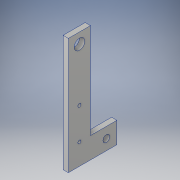
# Autodesk Inventor part: PaddleCollection2.1AxleSupport
Saved by Autodesk Inventor 2019 (Build 230136000, 136)
## iProperties
Created: 2018-10-20
Part Number: PaddleCollection2.1AxleSupport
Material: Aluminum 6061
Document SubType Name: Modeling
Designer: User
Density: 2.7 g/cm^3
Appearance: Aluminum - Flat
Author: User
Autodesk Inventor part; units mm, degrees
ref_plane "YZ Plane" through (0, 0, 0) normal (1, 0, 0) x (0, 1, 0)
ref_plane "XZ Plane" through (0, 0, 0) normal (0, 1, 0) x (-1, 0, 0)
ref_plane "XY Plane" through (0, 0, 0) normal (0, 0, 1) x (1, 0, 0)
sketch "Sketch1" plane through (0, 0, 0) normal (1, 0, 0) x (0, 1, 0)
  line L0 (0, 0) -> (139.7, 0)
  line L1 (139.7, 0) -> (139.7, -58.2676)
  line L2 (139.7, -58.2676) -> (0, -58.2676)
  line L3 (0, -58.2676) -> (0, 0)
  circle A0 centre (127, -13.2588) radius 6.35
  circle A1 centre (12.7, -45.5676) radius 4.064
  line L4 (139.7, -58.2676) -> (25.4, -58.2676)
  line L5 (25.4, -58.2676) -> (25.4, -26.5176)
  line L6 (25.4, -26.5176) -> (139.7, -26.5176)
  line L7 (139.7, -26.5176) -> (139.7, -58.2676)
  dimension "d0" = 139.7
  dimension "d2" = 12.7
  dimension "d3" = 8.128
  dimension "d5" = 114.3
  dimension "d6" = 12.7
  dimension "d7" = 12.7
  dimension "d8" = 13.2588
  dimension "d9" = 12.7
  dimension "d24" = 26.5176
  dimension "d26" = 32.3088
  constraints: 16 end point, 4 parallel, 2 centre point, 2 horizontal, 2 perpendicular
  measures "d0" distance of L1.end L2.end
  measures "d2" diameter of A0
  measures "d3" diameter of A1
  measures "d5" horizontal distance of A1.centre A0.centre
  measures "d6" distance from line of L2 A1.centre
  measures "d7" distance from line of L3 A1.centre
  measures "d8" distance from line of A0.centre L6
  measures "d9" distance from line of A1.centre L5
  measures "d24" distance between parallel lines of L0 L6
  measures "d26" vertical distance of A1.centre A0.centre
extrude "Extrusion1" add sketch "Sketch1" along normal blind 6.35 contours L0 L1 L6 L5 L2 L3
sketch "Sketch2" plane through (6.35, 0, 0) normal (1, 0, 0) x (0, 0, -1)
  line L0 (0, 0) -> (58.2676, 0) projected
  line L1 (26.5176, 139.7) -> (0, 139.7) projected
  line L2 (0, 139.7) -> (0, 0) projected
  point P0 (13.2588, 25.4)
  point P1 (13.2588, 63.5)
  dimension "d12" = 63.5
  dimension "d13" = 25.4
  dimension "d14" = 26.5176
  dimension "d15" = 13.2588
  dimension "d16" = 13.2588
  measures "d12" distance from line of L0 point (13.259, 63.5)
  measures "d13" distance from line of L0 point (13.259, 25.4)
  measures "d14" distance of L1.start L1.end
  measures "d15" distance from line of L2 point (13.259, 63.5)
  measures "d16" distance from line of L2 point (13.259, 25.4)
hole "Hole1" at (6.35, 25.4, -13.2588) at (6.35, 63.5, -13.2588) direction (-1, 0, 0) diameter 3.81 end through all
equation "\"d8\" = 0.5 * d24"
equation "\"d15\" = 0.5 * d14"
equation "\"d16\" = d15"
body "Solid1"
